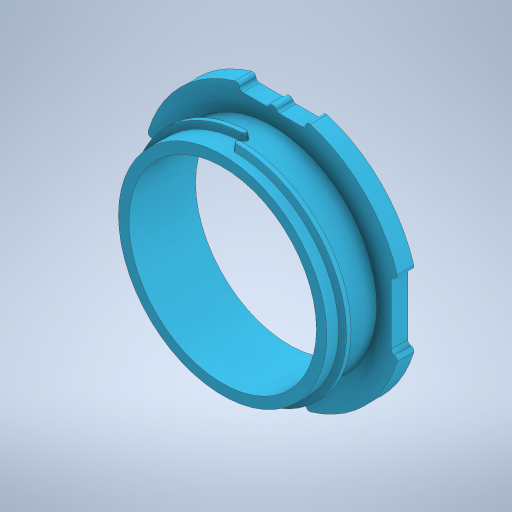
# Autodesk Inventor part: rosca_1
Saved by Autodesk Inventor 2023.2 (Build 272271030, 271C)
## iProperties
Created: 2023-10-23
Part Number: rosca_1
Material: Generic
Document SubType Name: Modeling
Designer: Cris Pat
Density: 1 g/cm^3
Appearance: Default
Author: Cris Pat
Autodesk Inventor part; units mm, degrees
ref_plane "YZ Plane" through (0, 0, 0) normal (1, 0, 0) x (0, 1, 0)
ref_plane "XZ Plane" through (0, 0, 0) normal (0, 1, 0) x (-1, 0, 0)
ref_plane "XY Plane" through (0, 0, 0) normal (0, 0, 1) x (1, 0, 0)
sketch "Sketch1" plane through (0, 0, 0) normal (0, 0, 1) x (1, 0, 0)
  circle A0 centre (0, 0) radius 31.2225
  dimension "d0" = 62.445
  constraints: 1 centre point, 1 coincident
  measures "d0" diameter of A0
extrude "Extrusion1" add sketch "Sketch1" along normal blind 4
sketch "Sketch2" plane through (0, 0, 4) normal (0, 0, 1) x (1, 0, 0)
  circle A0 centre (0, 0) radius 25
  dimension "d3" = 50
  constraints: 1 centre point, 1 coincident
  measures "d3" diameter of A0
extrude "Extrusion2" add sketch "Sketch2" along normal blind 12
sketch "Sketch3" plane through (0, 0, 0) normal (1, 0, 0) x (0, 1, 0)
  line L0 (31.2225, 4) -> (-31.2225, 4) construction
  line L1 (25, 4) -> (25, 16) construction
  line L2 (25, 10.944) -> (26.5, 10.556)
  line L3 (26.5, 10.556) -> (26.5, 9.444)
  line L4 (26.5, 9.444) -> (25, 9.056)
  line L5 (25, 9.056) -> (25, 10.944)
  point P0 (0, 0)
  point P1 (25.75, 10.75)
  point P2 (25.75, 9.25)
  point P3 (26.5, 10)
  dimension "d10" = 1.5
  dimension "d11" = 6
  dimension "d12" = 75.5
  dimension "d13" = 1.5
  constraints: 9 end point, 3 midpoint, 1 equal length, 1 parallel, 1 vertical, 1 vertical alignment
  measures "d10" distance of point (25.75, 10.75) point (25.75, 9.25)
  measures "d11" distance from line of L0 point (26.5, 10)
  measures "d12" angle of L5 L2
  measures "d13" distance between parallel lines of L5 L3
coil "Coil1" sketch "Sketch3" operation add axis through (0, 0, -10) along (0, 0, 1) pitch 3 turns 1 hand right
chamfer "Chamfer1" distance 0.7 angle 45 4 edges at (0, 25.75, 10.75) (0, 25.75, 9.25) (0, 25.75, 13.75) (0, 25.75, 12.25)
sketch "Sketch4" plane through (0, 0, 16) normal (0, 0, 1) x (1, 0, 0)
  circle A0 centre (0, 0) radius 22.5
  dimension "d25" = 45
  constraints: 1 centre point, 1 coincident
  measures "d25" diameter of A0
extrude "Extrusion3" cut sketch "Sketch4" against normal through all
sketch "Sketch5" plane through (0, 0, 4) normal (0, 0, 1) x (1, 0, 0)
  line L0 (-8, 31.2225) -> (8, 31.2225)
  line L1 (8, 31.2225) -> (8, 28.3945)
  line L2 (8, 28.3945) -> (-8, 28.3945)
  line L3 (-8, 28.3945) -> (-8, 31.2225)
  circle A0 centre (0, 0) radius 29.5 construction
  circle A1 centre (0, 0) radius 31.2225 construction
  point P0 (0, 31.2225)
  dimension "d28" = 59
  dimension "d29" = 16
  constraints: 8 end point, 2 parallel, 1 coincident, 1 horizontal, 1 midpoint, 1 perpendicular, 1 tangent, 1 vertical alignment, 3 other
  measures "d29" distance between parallel lines of L1 L3
extrude "Extrusion4" cut sketch "Sketch5" against normal through all
fillet "Fillet1" radius 0.8 4 edges at (-8, 30.1802, 2) (-8, 28.3945, 2) (8, 30.1802, 2) (8, 28.3945, 2)
pattern_circular "Circular Pattern1" count 4 over 360 about axis through (0, 0, 10.556) along (0, 0, 1) of "Fillet1", "Extrusion4"
sketch "Sketch6" plane through (0, 0, 0) normal (0, 0, 1) x (1, 0, 0)
  line L0 (7.2016, 28.3945) -> (-7.2016, 28.3945) construction
  arc A0 (1, 28.3945) -> (-1, 28.3945) centre (0, 28.3945) ccw
  line L1 (1, 28.3945) -> (-1, 28.3945)
  point P0 (0, 0)
  dimension "d36" = 1
  constraints: 2 end point, 2 point on circle, 2 point on line, 1 centre point, 1 horizontal, 1 midpoint, 1 vertical alignment
  measures "d36" radius of A0
extrude "Extrusion5" add sketch "Sketch6" along normal up to surface (4 mm away)
fillet "Fillet2" radius 0.8 2 edges at (1, 28.3945, 2) (-1, 28.3945, 2)
body "Solid1"
